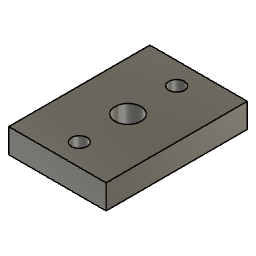
전방 덮개 브라켓2 (Autodesk Fusion 360 design; units mm, degrees)
Autodesk Fusion 360 part; units mm, degrees
sketch "스케치1" plane through (0, 0, 0) normal (0, 0, 1) x (1, 0, 0)
  line L0 (10, 14.5) -> (-10, 14.5)
  line L1 (-10, 14.5) -> (-10, -14.5)
  line L2 (-10, -14.5) -> (10, -14.5)
  line L3 (10, -14.5) -> (10, 14.5)
  line L4 (10, 14.5) -> (-10, -14.5) construction
  line L5 (-10, 14.5) -> (10, -14.5) construction
  circle A0 centre (0, 0) radius 2.65
  line L6 (0, 0) -> (0, 10)
  circle A1 centre (0, 10) radius 1.6
  line L7 (0, 0) -> (0, -10)
  circle A2 centre (0, -10) radius 1.6
  dimension "d1" = 20
  dimension "d2" = 29
  dimension "d3" = 5.3
  dimension "d4" = 10
  dimension "d5" = 3.2
  dimension "d6" = 10
  dimension "d7" = 3.2
  constraint horizontal L0
  constraint perpendicular L0 L1
  constraint parallel L0 L2
  constraint parallel L1 L3
  constraint coincident L4 A0.centre
  constraint coincident L5 A0.centre
  constraint coincident A0.centre L6.start
  constraint vertical L6
  constraint coincident L6.end A1.centre
  constraint parallel L6 L7
  constraint coincident L7.end A2.centre
  measures "d1" distance of L1.end L2.end
  measures "d2" distance of L0.end L1.end
  measures "d3" diameter of A0
  measures "d4" distance of A0.centre L6.end
  measures "d5" diameter of A1
  measures "d6" distance of A0.centre L7.end
  measures "d7" diameter of A2
extrude "돌출1" add sketch "스케치1" along normal blind 5
extrude "돌출2" add sketch "스케치1" along normal blind 2.8 contours A1 | A2
